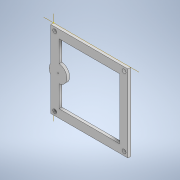
# Autodesk Inventor part: P1
Saved by Autodesk Inventor 2022 (Build 260153000, 153)
## iProperties
Created: 2022-11-21
Part Number: P1
Material: Genérico
Document SubType Name: Modeling
Designer: javie
Density: 1 g/cm^3
Appearance: Valor por defecto
Autodesk Inventor part; units mm, degrees
ref_plane "YZ Plane" through (0, 0, 0) normal (1, 0, 0) x (0, 1, 0)
ref_plane "XZ Plane" through (0, 0, 0) normal (0, 1, 0) x (-1, 0, 0)
ref_plane "XY Plane" through (0, 0, 0) normal (0, 0, 1) x (1, 0, 0)
sketch "Boceto1" plane through (0, 0, 0) normal (0, 0, 1) x (1, 0, 0)
  point P0 (0, 0)
sketch "0" plane through (0, 0, 0) normal (0, 0, 1) x (1, 0, 0)
  circle A0 centre (-671.6471, -277.2868) radius 3.5
  circle A1 centre (-545.6471, -277.2868) radius 3.5
  circle A2 centre (-671.6471, -403.2868) radius 3.5
  circle A3 centre (-545.6471, -403.2868) radius 3.5
  circle A4 centre (7, -133) radius 3.5
  circle A5 centre (7, -7) radius 3.5
  circle A6 centre (133, -133) radius 3.5
  circle A7 centre (133, -7) radius 3.5
  circle A8 centre (-670.5803, -255.684) radius 3.5
  circle A9 centre (-670.5803, -129.684) radius 3.5
  circle A10 centre (-544.5803, -255.684) radius 3.5
  circle A11 centre (-544.5803, -129.684) radius 3.5
  circle A12 centre (-741.4316, -468.1442) radius 3.5
  circle A13 centre (-799.8971, -377.5076) radius 3.5
  line L0 (-840.9891, -326.5002) -> (-840.9891, -274.8276)
  line L1 (-840.9891, -274.8276) -> (-825.9891, -274.8276)
  line L2 (-825.9891, -274.8276) -> (-825.9891, -319.9531)
  circle A14 centre (-833.7364, -286.5276) radius 3.5
  line L3 (-553.6471, -387.9066) -> (-553.6471, -402.2868)
  line L4 (-553.6471, -402.2868) -> (-663.6471, -402.2868)
  line L5 (-663.6471, -402.2868) -> (-663.6471, -388.2868)
  line L6 (-663.6471, -388.2868) -> (-663.6471, -356.1613)
  arc A15 (-681.67, -501.8739) -> (-685.67, -501.8739) centre (-683.67, -501.8739) ccw
  line L7 (-681.67, -501.8739) -> (-681.67, -539.0536)
  arc A16 (-685.67, -539.0536) -> (-681.67, -539.0536) centre (-683.67, -539.0536) ccw
  line L8 (-685.67, -539.0536) -> (-685.67, -501.8739)
  line L9 (-585.2407, -487.858) -> (-585.2407, -480.358)
  line L10 (-585.2407, -480.358) -> (-669.2108, -480.358)
  arc A17 (-671.9229, -479.9831) -> (-669.2108, -480.358) centre (-669.2108, -470.358) ccw
  line L11 (-671.9229, -479.9831) -> (-696.1106, -473.1676)
  arc A18 (-696.1106, -473.1676) -> (-698.0161, -472.8254) centre (-698.8228, -482.7928) ccw
  arc A19 (-699.9334, -472.4798) -> (-698.0161, -472.8254) centre (-697.2095, -462.858) ccw
  line L12 (-766.1674, -437.2692) -> (-728.9877, -437.2692)
  arc A20 (-728.9877, -437.2692) -> (-728.9877, -433.2692) centre (-728.9877, -435.2692) ccw
  line L13 (-728.9877, -433.2692) -> (-766.1674, -433.2692)
  arc A21 (-766.1674, -433.2692) -> (-766.1674, -437.2692) centre (-766.1674, -435.2692) ccw
  line L14 (-677.5803, -183.3567) -> (-677.5803, -122.684)
  line L15 (-677.5803, -122.684) -> (-537.5803, -122.684)
  line L16 (-537.5803, -122.684) -> (-537.5803, -262.684)
  line L17 (-537.5803, -262.684) -> (-677.5803, -262.684)
  line L18 (-677.5803, -262.684) -> (-677.5803, -202.0114)
  line L19 (-662.5803, -208.5585) -> (-662.5803, -247.684)
  line L20 (-662.5803, -247.684) -> (-552.5803, -247.684)
  line L21 (-552.5803, -247.684) -> (-552.5803, -137.684)
  line L22 (-552.5803, -137.684) -> (-662.5803, -137.684)
  line L23 (-662.5803, -137.684) -> (-662.5803, -176.8095)
  line L24 (0, -60.6726) -> (0, 0)
  line L25 (0, 0) -> (140, 0)
  line L26 (140, 0) -> (140, -140)
  line L27 (140, -140) -> (0, -140)
  line L28 (0, -140) -> (0, -79.3274)
  line L29 (15, -85.8745) -> (15, -125)
  line L30 (15, -125) -> (125, -125)
  line L31 (125, -125) -> (125, -15)
  line L32 (125, -15) -> (15, -15)
  line L33 (15, -15) -> (15, -54.1255)
  circle A22 centre (-545.752, -549.8856) radius 3.5
  line L34 (-652.1152, -541.8856) -> (-553.752, -541.8856)
  line L35 (-553.752, -541.8856) -> (-553.752, -502.7601)
  line L36 (-652.1152, -556.8856) -> (-652.1152, -541.8856)
  line L37 (-652.1152, -416.8856) -> (-538.752, -416.8856)
  line L38 (-538.752, -416.8856) -> (-538.752, -477.5582)
  line L39 (-652.1152, -431.8856) -> (-652.1152, -416.8856)
  circle A23 centre (-545.752, -423.8856) radius 3.5
  arc A24 (0, -60.6726) -> (0, -79.3274) centre (13, -70) ccw
  arc A25 (-677.5803, -183.3567) -> (-677.5803, -202.0114) centre (-664.5803, -192.684) ccw
  arc A26 (-840.9891, -326.5002) -> (-840.9891, -345.155) centre (-827.9891, -335.8276) ccw
  arc A27 (-678.6471, -330.9594) -> (-678.6471, -349.6141) centre (-665.6471, -340.2868) ccw
  arc A28 (-804.8971, -395.9384) -> (-795.5615, -419.0058) centre (-790.9049, -403.6985) ccw
  arc A29 (-553.752, -471.0111) -> (-553.752, -502.7601) centre (-551.752, -486.8856) ccw
  arc A30 (-731.011, -479.8384) -> (-703.3644, -487.858) centre (-715.2407, -477.1364) ccw
  arc A31 (15, -85.8745) -> (15, -54.1255) centre (13, -70) ccw
  arc A32 (-662.5803, -208.5585) -> (-662.5803, -176.8095) centre (-664.5803, -192.684) ccw
  line L40 (-804.8971, -395.9384) -> (-804.8971, -370.5076)
  line L41 (-804.8971, -370.5076) -> (-789.903, -370.5076)
  line L42 (-789.903, -370.5076) -> (-789.903, -382.3505)
  arc A33 (-789.903, -382.3505) -> (-788.2029, -387.9282) centre (-779.903, -382.3505) ccw
  line L43 (-780.1834, -415.5748) -> (-780.1834, -420.3477)
  arc A34 (-780.1834, -420.3477) -> (-779.8086, -423.0599) centre (-770.1834, -420.3477) ccw
  line L44 (-779.8086, -423.0599) -> (-777.4954, -431.2692)
  line L45 (-777.4954, -431.2692) -> (-725.4954, -431.2692)
  arc A35 (-725.4954, -439.2692) -> (-725.4954, -431.2692) centre (-725.2393, -435.2692) ccw
  line L46 (-725.4954, -439.2692) -> (-775.2411, -439.2692)
  line L47 (-775.2411, -439.2692) -> (-773.0582, -447.0163)
  arc A36 (-772.6834, -449.7284) -> (-773.0582, -447.0163) centre (-782.6834, -449.7284) ccw
  line L48 (-772.6834, -449.7284) -> (-772.6834, -533.6985)
  line L49 (-772.6834, -533.6985) -> (-787.6834, -533.6985)
  line L50 (-787.6834, -533.6985) -> (-787.6834, -449.7284)
  arc A37 (-787.6834, -449.7284) -> (-788.0582, -447.0163) centre (-797.6834, -449.7284) ccw
  line L51 (-788.0582, -447.0163) -> (-794.8737, -422.8286)
  arc A38 (-795.216, -420.9231) -> (-794.8737, -422.8286) centre (-785.2486, -420.1164) ccw
  arc A39 (-795.216, -420.9231) -> (-795.5615, -419.0058) centre (-805.1834, -421.7297) ccw
  arc A40 (-780.1834, -415.5748) -> (-788.2029, -387.9282) centre (-790.9049, -403.6985) ccw
  line L52 (-663.6471, -324.4123) -> (-663.6471, -278.2868)
  line L53 (-663.6471, -278.2868) -> (-553.6471, -278.2868)
  line L54 (-553.6471, -278.2868) -> (-553.6471, -331.7868)
  line L55 (-553.6471, -331.7868) -> (-538.6471, -331.7868)
  line L56 (-538.6471, -331.7868) -> (-538.6471, -270.2868)
  line L57 (-538.6471, -270.2868) -> (-678.6471, -270.2868)
  line L58 (-678.6471, -270.2868) -> (-678.6471, -330.9594)
  line L59 (-678.6471, -349.6141) -> (-678.6471, -410.2868)
  line L60 (-678.6471, -410.2868) -> (-538.6471, -410.2868)
  line L61 (-538.6471, -410.2868) -> (-538.6471, -348.7868)
  line L62 (-538.6471, -348.7868) -> (-553.6471, -348.7868)
  line L63 (-553.6471, -348.7868) -> (-553.6471, -388.2868)
  arc A41 (-663.6471, -356.1613) -> (-663.6471, -324.4123) centre (-665.6471, -340.2868) ccw
  line L64 (-813.8558, -328.3276) -> (-690.9891, -328.3276)
  line L65 (-690.9891, -328.3276) -> (-690.9891, -343.3276)
  line L66 (-690.9891, -343.3276) -> (-813.8558, -343.3276)
  line L67 (-825.9891, -351.7021) -> (-825.9891, -396.8276)
  line L68 (-825.9891, -396.8276) -> (-840.9891, -396.8276)
  line L69 (-840.9891, -396.8276) -> (-840.9891, -345.155)
  arc A42 (-825.9891, -351.7021) -> (-813.8558, -343.3276) centre (-827.9891, -335.8276) ccw
  arc A43 (-813.8558, -328.3276) -> (-825.9891, -319.9531) centre (-827.9891, -335.8276) ccw
  line L70 (-538.752, -496.213) -> (-538.752, -556.8856)
  line L71 (-538.752, -556.8856) -> (-652.1152, -556.8856)
  line L72 (-553.752, -471.0111) -> (-553.752, -431.8856)
  line L73 (-553.752, -431.8856) -> (-652.1152, -431.8856)
  arc A44 (-538.752, -496.213) -> (-538.752, -477.5582) centre (-551.752, -486.8856) ccw
  line L74 (-703.3644, -487.858) -> (-698.5915, -487.858)
  arc A45 (-695.8793, -488.2328) -> (-698.5915, -487.858) centre (-698.5915, -497.858) ccw
  line L75 (-695.8793, -488.2328) -> (-687.67, -490.546)
  line L76 (-687.67, -490.546) -> (-687.67, -542.546)
  arc A46 (-687.67, -542.546) -> (-679.67, -542.546) centre (-683.67, -542.8021) ccw
  line L77 (-679.67, -542.546) -> (-679.67, -492.8002)
  line L78 (-679.67, -492.8002) -> (-671.9229, -494.9831)
  arc A47 (-671.9229, -494.9831) -> (-669.2108, -495.358) centre (-669.2108, -485.358) ccw
  line L79 (-669.2108, -495.358) -> (-585.2407, -495.358)
  line L80 (-585.2407, -495.358) -> (-585.2407, -480.358)
  line L81 (-723.0008, -463.1442) -> (-748.4316, -463.1442)
  line L82 (-748.4316, -463.1442) -> (-748.4316, -478.1383)
  line L83 (-748.4316, -478.1383) -> (-736.5887, -478.1383)
  arc A48 (-731.011, -479.8384) -> (-736.5887, -478.1383) centre (-736.5887, -488.1383) ccw
  arc A49 (-699.9334, -472.4798) -> (-723.0008, -463.1442) centre (-715.2407, -477.1364) ccw
  line L84 (-855.7327, -108.1134) -> (-523.7327, -108.1134)
  line L85 (-523.7327, -108.1134) -> (-523.7327, -571.1134)
  line L86 (-523.7327, -571.1134) -> (-855.7327, -571.1134)
  line L87 (-855.7327, -571.1134) -> (-855.7327, -108.1134)
  circle A50 centre (13, -70) radius 1
  dimension "d11" = 2
  constraints: 176 end point, 66 point on circle, 51 centre point, 1 coincident
  measures "d11" diameter of A50
extrude "Extrusión1" add sketch "0" along normal blind 5 contours L24 L25 L26 L27 L28 A24
